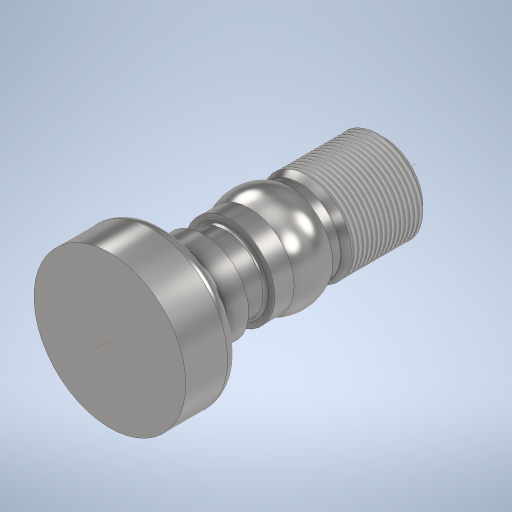
# Autodesk Inventor part: W4
Saved by Autodesk Inventor 2023 (Build 270158000, 158)
## iProperties
Created: 2023-01-07
Part Number: W4
Material: Stal, miękka
Document SubType Name: Modeling
Designer: mkhamenk
Density: 7.85 g/cm^3
Appearance: Częściowo polerowany
Mass: 4160.82 g
Surface Area: 605.754 cm^2
Volume: 530.041 cm^3
Author: mkhamenk
Autodesk Inventor part; units mm, degrees
ref_plane "XZ Plane" through (0, 0, 0) normal (0, 1, 0) x (-1, 0, 0)
ref_plane "XY Plane" through (0, 0, 0) normal (0, 0, 1) x (1, 0, 0)
sketch "Szkic1" plane through (0, 0, 0) normal (0, 0, 1) x (1, 0, 0)
  circle A0 centre (0, 0) radius 49
  dimension "d0" = 98
  constraints: 1 centre point, 1 coincident
  measures "d0" diameter of A0
extrude "Wyciągnięcie proste1" add sketch "Szkic1" against normal blind 35
sketch "Szkic2" plane through (0, 0, -35) normal (0, 0, -1) x (-1, 0, 0)
  circle A0 centre (0, 0) radius 29
  circle A1 centre (0, 0) radius 49 projected
  dimension "d3" = 58
  constraints: 1 centre point, 1 concentric
  measures "d3" diameter of A0
extrude "Wyciągnięcie proste2" add sketch "Szkic2" along normal blind 55 contours A0
fillet "Zaokrąglenie1" radius 8 1 edges at (-49, 0, -35)
fillet "Zaokrąglenie2" radius 12 1 edges at (29, 0, -35)
ref_plane "Płaszczyzna konstrukcyjna1" through (0, 0, -35) normal (0, -1, 0) x (0, 0, -1)
sketch "Szkic3" plane through (0, 0, -35) normal (0, -1, 0) x (0, 0, -1)
  line L0 (12, -29) -> (55, -29) projected
  line L1 (55, -29) -> (55, 29) projected
  line L2 (55, -29) -> (80, -29) construction
  line L3 (67.5, -32.202) -> (67.5, 45.2604) construction
  arc A0 (55, -29) -> (80, -29) centre (67.5, -6.202) ccw
  line L4 (80, -29) -> (80, 0)
  line L5 (80, 0) -> (55, 0)
  point P0 (-35, 0)
  dimension "d9" = 25
  dimension "d10" = 12.5
  dimension "d11" = 26
  constraints: 8 end point, 3 point on circle, 2 vertical, 1 centre point, 1 midpoint, 1 point on line
  measures "d9" distance of L0.end L2.end
  measures "d10" distance between parallel lines of L1 L3
  measures "d11" radius of A0
revolve "Obrót1" add sketch "Szkic3" angle 360 about axis through (0, 0, -115) along (0, 0, 1)
sketch "Szkic4" plane through (0, 0, -115) normal (0, 0, -1) x (-1, 0, 0)
  circle A0 centre (0, 0) radius 29 projected
extrude "Wyciągnięcie proste3" add sketch "Szkic4" along normal blind 62
sketch "Szkic5" plane through (0, 0, -35) normal (0, -1, 0) x (0, 0, -1)
  line L0 (12, 29) -> (55, 29) projected
  line L1 (34, 66.9437) -> (34, -72.7347) construction
  line L2 (142, -29) -> (142, 29) projected
  line L3 (25.6184, 29) -> (26.5, 24)
  line L4 (26.5, 24) -> (41.5, 24)
  line L5 (41.5, 24) -> (42.3816, 29)
  line L6 (-70.4, 0) -> (177.4, 0) projected
  point P0 (-35, 0)
  dimension "d15" = 108
  dimension "d16" = 5
  dimension "d17" = 7.5
  dimension "d18" = 15
  dimension "d19" = 10
  constraints: 8 end point, 2 point on line, 1 equal length, 1 horizontal, 1 vertical
  measures "d15" distance between parallel lines of L1 L2
  measures "d16" distance from line of L0 L3.end
  measures "d17" distance from line of L1 L3.end
  measures "d18" distance of L3.end L4.end
  measures "d19" angle of L1 L3
revolve "Obrót2" cut sketch "Szkic5" angle 360 about axis through (0, 0, -35) along (0, 0, -1)
fillet "Zaokrąglenie3" radius 2 1 edges at (-24, 0, -76.5)
fillet "Zaokrąglenie4" radius 2 1 edges at (-24, 0, -61.5)
sketch "Szkic6" plane through (0, 0, -35) normal (0, -1, 0) x (0, 0, -1)
  line L0 (80, 29) -> (142, 29) projected
  line L1 (80, 29) -> (80, -29) projected
  line L2 (80, 29) -> (142, 29) projected
  line L3 (80, 26.5) -> (87.6699, 26.5)
  line L4 (87.6699, 26.5) -> (92, 29)
  line L5 (-70.4, 0) -> (177.4, 0) projected
  point P0 (-35, 0)
  point P1 (83.8349, 26.5)
  dimension "d23" = 2.5
  dimension "d24" = 30
  dimension "d25" = 12
  constraints: 4 end point, 2 point on line, 1 horizontal, 1 midpoint
  measures "d23" distance from line of L0 point (83.835, 26.5)
  measures "d24" angle of L0 L4
  measures "d25" distance of L0.start L4.end
revolve "Obrót3" cut sketch "Szkic6" angle 360 about axis through (0, 0, -35) along (0, 0, -1)
fillet "Zaokrąglenie5" radius 0.8 1 edges at (-26.5, 0, -115)
fillet "Zaokrąglenie6" radius 0.8 1 edges at (-26.5, 0, -122.6699)
chamfer "Faza1" distance 4 angle 45 1 edges at (29, 0, -177)
thread "Gwint1" size "M58x3" class "6g" standard "ANSI Metric M Profile" full length
sketch "Szkic10" plane through (0, 0, -177) normal (0, 0, -1) x (-1, 0, 0)
  circle A0 centre (0, 0) radius 25 projected
  constraints: 1 coincident
hole "Otwór3" at (0, 0, -177) direction (0, 0, 1) diameter 16 depth 100 tip angle 118
sketch "Szkic11" plane through (0, 0, -177) normal (0, 0, -1) x (-1, 0, 0)
  circle A0 centre (0, 0) radius 25 projected
  constraints: 1 coincident
hole "Otwór4" at (0, 0, -177) direction (0, 0, 1) diameter 40 depth 50
sketch "Szkic12" plane through (0, 0, -35) normal (0, -1, 0) x (0, 0, -1)
  line L0 (42, -8) -> (92, -8) projected
  line L1 (92, -20) -> (142, -20) projected
  line L2 (92, -20) -> (92, 20) projected
  arc A0 (59.5038, -8) -> (92, -20) centre (92, 30) ccw
  line L3 (-70.4, 0) -> (177.4, 0) projected
  point P0 (-35, 0)
  dimension "d64" = 50
  constraints: 2 point on circle, 1 centre point, 1 point on line, 1 tangent
  measures "d64" radius of A0
revolve "Obrót5" cut sketch "Szkic12" angle 360 about axis through (0, 0, -35) along (0, 0, -1)
fillet "Zaokrąglenie7" radius 10 2 edges at (5.6569, -5.6569, -94.5038) (-5.6569, 5.6569, -94.5038)
chamfer "Faza2" distance 37 angle 5 1 edges at (0, -20, -177) measured on face at (0, -20, -176.5)
